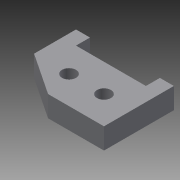
# Autodesk Inventor part: P1-3
Saved by Autodesk Inventor 2014 (Build 180170000, 170)
## iProperties
Created: 2017-02-06
Part Number: P1-3
Material: Generic
Document SubType Name: Modeling
Designer: mschaffel
Density: 1 g/cm^3
Appearance: Default
Author: mschaffel
Autodesk Inventor part; units mm, degrees
ref_plane "YZ Plane" through (0, 0, 0) normal (1, 0, 0) x (0, 1, 0)
ref_plane "XZ Plane" through (0, 0, 0) normal (0, 1, 0) x (-1, 0, 0)
ref_plane "XY Plane" through (0, 0, 0) normal (0, 0, 1) x (1, 0, 0)
sketch "Sketch1" plane through (0, 0, 0) normal (0, 1, 0) x (-1, 0, 0)
  line L0 (0, 0) -> (0, 63.5)
  line L1 (0, 63.5) -> (50.8, 63.5)
  line L2 (0, 0) -> (12.7, 0)
  line L3 (12.7, 0) -> (12.7, 12.7)
  line L4 (12.7, 12.7) -> (76.2, 12.7)
  line L5 (76.2, 12.7) -> (76.2, 0)
  line L6 (76.2, 0) -> (88.9, 0)
  line L7 (88.9, 0) -> (88.9, 38.1)
  line L8 (88.9, 38.1) -> (50.8, 63.5)
  circle A0 centre (25.4, 38.1) radius 6.35
  circle A1 centre (57.15, 38.1) radius 6.35
  dimension "d0" = 63.5
  dimension "d1" = 50.8
  dimension "d2" = 63.5
  dimension "d3" = 12.7
  constraints: 18 end point, 3 parallel, 2 centre point, 2 perpendicular, 1 collinear, 1 vertical
  measures "d0" distance of L0.start L0.end
  measures "d1" distance of L0.end L1.end
  measures "d2" distance of L3.end L4.end
  measures "d3" diameter of A0
extrude "Extrusion1" add sketch "Sketch1" along normal blind 19.05
body "Solid1"
